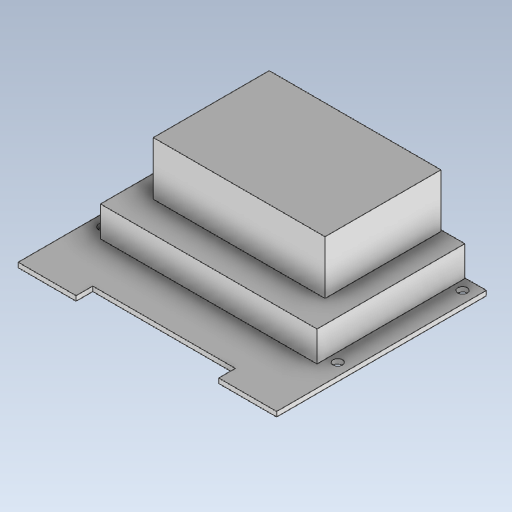
# Autodesk Inventor part: JetsonXavierNX_and_EN715
Saved by Autodesk Inventor 2020 (Build 240168000, 168)
## iProperties
Part Number: JetsonXavierNX_and_EN715
Material: 一般
Document SubType Name: Modeling
Designer: Masato Kubotera
Density: 1 g/cm^3
Appearance: 既定
Description: ReadyMade
Mass: 97.5955 g
Surface Area: 209.001 cm^2
Volume: 97.5955 cm^3
Author: Masato Kubotera
Autodesk Inventor part; units mm, degrees
ref_plane "YZ Plane" through (0, 0, 0) normal (1, 0, 0) x (0, 1, 0)
ref_plane "XZ Plane" through (0, 0, 0) normal (0, 1, 0) x (-1, 0, 0)
ref_plane "XY Plane" through (0, 0, 0) normal (0, 0, 1) x (1, 0, 0)
sketch "スケッチ1" plane through (0, 0, 0) normal (0, 0, 1) x (1, 0, 0)
  line L0 (35.3, 43.5) -> (-35.3, 43.5)
  line L1 (-35.3, 43.5) -> (-35.3, -43.5)
  line L2 (-35.3, -43.5) -> (35.3, -43.5)
  line L3 (35.3, 43.5) -> (-35.3, -43.5) construction
  line L4 (-35.3, 43.5) -> (35.3, -43.5) construction
  circle A0 centre (-31.3, -39.5) radius 1.6
  circle A1 centre (10.7, -39.5) radius 1.6
  line L5 (29.7, 0) -> (-35.3, 0) construction
  circle A2 centre (-31.3, 39.5) radius 1.6
  circle A3 centre (10.7, 39.5) radius 1.6
  line L6 (14.65, 36.45) -> (-35.1, 36.45)
  line L7 (-35.1, 36.45) -> (-35.1, -36.45)
  line L8 (-35.1, -36.45) -> (14.65, -36.45)
  line L9 (14.65, -36.45) -> (14.65, 36.45)
  line L10 (14.65, 36.45) -> (-35.1, -36.45) construction
  line L11 (-35.1, 36.45) -> (14.65, -36.45) construction
  line L12 (35.3, -24) -> (29.7, -24)
  line L13 (29.7, -24) -> (29.7, 24)
  line L14 (29.7, 24) -> (35.3, 24)
  line L15 (35.3, -43.5) -> (35.3, -24)
  line L16 (35.3, 24) -> (35.3, 43.5)
  line L17 (4.4, 28.9) -> (-34.6, 28.9)
  line L18 (-34.6, 28.9) -> (-34.6, -28.9)
  line L19 (-34.6, -28.9) -> (4.4, -28.9)
  line L20 (4.4, -28.9) -> (4.4, 28.9)
  line L21 (4.4, 28.9) -> (-34.6, -28.9) construction
  line L22 (-34.6, 28.9) -> (4.4, -28.9) construction
  line L23 (-35.3, 11.2) -> (-12.8, 11.2)
  line L24 (-12.8, 11.2) -> (-12.8, 28)
  line L25 (-12.8, 28) -> (-35.3, 28)
  line L26 (-35.3, 11.2) -> (-37.8, 11.2)
  line L27 (-37.8, 11.2) -> (-37.8, 28)
  line L28 (-37.8, 28) -> (-35.3, 28)
  line L29 (-36.3, 7.17) -> (-19.3, 7.17)
  line L30 (-19.3, 7.17) -> (-19.3, -5.93)
  line L31 (-19.3, -5.93) -> (-36.3, -5.93)
  line L32 (-36.3, -5.93) -> (-36.3, 7.17)
  line L33 (-36.3, -12.41) -> (-25.3, -12.41)
  line L34 (-25.3, -12.41) -> (-25.3, -28.01)
  line L35 (-25.3, -28.01) -> (-36.3, -28.01)
  line L36 (-36.3, -28.01) -> (-36.3, -12.41)
  point P0 (0, 0)
  point P1 (-10.225, 0)
  point P2 (-10.225, 0)
  point P3 (-15.1, 0)
  dimension "d0" = 70.6
  dimension "d1" = 87
  dimension "d2" = 3.2
  dimension "d3" = 3.2
  dimension "d4" = 4
  dimension "d5" = 46
  dimension "d6" = 4
  dimension "d7" = 4
  dimension "d8" = 49.75
  dimension "d9" = 72.9
  dimension "d10" = 0.2
  dimension "d11" = 19.5
  dimension "d12" = 5.6
  dimension "d13" = 39
  dimension "d14" = 57.8
  dimension "d15" = 7.55
  dimension "d16" = 0.5
  dimension "d23" = 22.5
  dimension "d24" = 16.8
  dimension "d26" = 2.5
  dimension "d27" = 13.1
  dimension "d28" = 16
  dimension "d29" = 1
  dimension "d37" = 11
  dimension "d38" = 15.6
  dimension "d42" = 15.5
  dimension "d43" = 4.03
  dimension "d44" = 6.48
  constraints: 74 end point, 11 parallel, 11 perpendicular, 9 midpoint, 8 horizontal, 4 centre point, 4 point on line, 3 collinear, 2 symmetric about line, 3 other
  measures "d0" distance of L2.end L1.end
  measures "d1" distance of L1.end L0.end
  measures "d2" diameter of A0
  measures "d3" diameter of A1
  measures "d4" distance from line of A0.centre L1
  measures "d5" distance from line of L1 A1.centre
  measures "d6" distance from line of L2 A0.centre
  measures "d7" distance from line of L2 A1.centre
  measures "d8" distance of L8.end L7.end
  measures "d9" distance of L7.end L6.end
  measures "d10" distance between parallel lines of L1 L7
  measures "d11" distance between parallel lines of L2 L12
  measures "d12" distance of L12.start L12.end
  measures "d13" distance of L19.end L18.end
  measures "d14" distance of L18.end L17.end
  measures "d15" distance between parallel lines of L8 L19
  measures "d16" distance between parallel lines of L18 L7
  measures "d23" distance of L24.end L25.end
  measures "d24" distance of L23.end L24.end
  measures "d26" distance of L27.end L25.end
  measures "d27" distance of L31.end L29.start
  measures "d28" distance between parallel lines of L30 L1
  measures "d29" distance between parallel lines of L32 L1
  measures "d37" distance of L33.start L33.end
  measures "d38" distance of L33.end L34.end
  measures "d42" distance between parallel lines of L0 L25
  measures "d43" distance between parallel lines of L23 L29
  measures "d44" distance between parallel lines of L33 L31
extrude "押し出し1" add sketch "スケッチ1" along normal blind 1.6 contours L16 L14 L13 L12 L15 L2 L1 L35 L7 L8 L9 L6 L25 L0 | L25 L7 L23 L1 | L23 L7 L29 L1 | L25 L18 L23 L7 | L7 L6 L9 L8 L35 L18 L19 L20 L17 L25 | L29 L7 L31 L1 | L23 L18 L29 L7 | L25 L24 L23 L18 | L18 L17 L20 L19 L35 L34 L33 L31 L30 L29 L23 L24 L25 | L31 L7 L33 L1 | L29 L18 L31 L7 | L33 L7 L35 L1 | L31 L18 L33 L7 | L29 L30 L31 L18 | L33 L18 L35 L7 | L33 L34 L35 L18
extrude "押し出し2" add sketch "スケッチ1" along normal blind 11.79 contours L25 L18 L23 L7 | L7 L6 L9 L8 L35 L18 L19 L20 L17 L25 | L23 L18 L29 L7 | L25 L24 L23 L18 | L18 L17 L20 L19 L35 L34 L33 L31 L30 L29 L23 L24 L25 | L29 L18 L31 L7 | L31 L18 L33 L7 | L29 L30 L31 L18 | L33 L18 L35 L7 | L33 L34 L35 L18
extrude "押し出し3" add sketch "スケッチ1" along normal blind 29.79 contours L25 L24 L23 L18 | L18 L17 L20 L19 L35 L34 L33 L31 L30 L29 L23 L24 L25 | L29 L30 L31 L18 | L33 L34 L35 L18
extrude "押し出し4" add sketch "スケッチ1" against normal blind 14.5 contours L25 L7 L23 L1 | L1 L26 L27 L28 | L25 L18 L23 L7 | L25 L24 L23 L18
extrude "押し出し5" add sketch "スケッチ1" against normal blind 16 contours L29 L7 L31 L1 | L1 L31 L32 L29 | L29 L18 L31 L7 | L29 L30 L31 L18
extrude "押し出し6" add sketch "スケッチ1" against normal blind 6.2 contours L33 L7 L35 L1 | L1 L35 L36 L33 | L33 L18 L35 L7 | L33 L34 L35 L18
equation "\"d7\" = d6"
